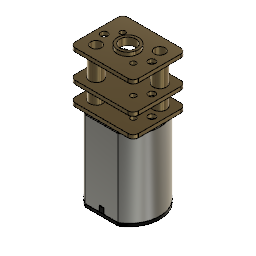
Semana4_Desafio2 v1 (Autodesk Fusion 360 design; units mm, degrees)
Autodesk Fusion 360 part; units mm, degrees
sketch "Sketch1" plane through (0, 0, 0) normal (0, 0, 1) x (1, 0, 0)
  line L0 (5, -5) -> (-5, -5)
  line L1 (-6, -4) -> (-6, 4)
  line L2 (-5, 5) -> (5, 5)
  line L3 (6, 4) -> (6, -4)
  line L4 (6, -5) -> (-6, 5) construction
  line L5 (-6, -5) -> (6, 5) construction
  circle A0 centre (0, 0) radius 2
  circle A1 centre (0, 0) radius 1.5
  circle A2 centre (-4.5, 0) radius 0.65
  circle A3 centre (4.5, 0) radius 0.65
  line L6 (-1.118, 1) -> (1.118, 1)
  arc A4 (-5, 5) -> (-6, 4) centre (-5, 4) ccw
  arc A5 (6, 4) -> (5, 5) centre (5, 4) ccw
  arc A6 (5, -5) -> (6, -4) centre (5, -4) ccw
  arc A7 (-6, -4) -> (-5, -5) centre (-5, -4) ccw
  point P0 (0, -1.5)
  dimension "d1" = 12
  dimension "d2" = 10
  dimension "d3" = 4
  dimension "d4" = 3
  dimension "d6" = 2.5
  dimension "d7" = 1.3
  dimension "d8" = 1.3
  dimension "d9" = 4.5
  dimension "d10" = 4.5
  dimension "d11" = 1
  dimension "d12" = 1
  dimension "d13" = 1
  dimension "d14" = 1
  constraint horizontal L0
  constraint perpendicular L0 L1
  constraint parallel L0 L2
  constraint parallel L1 L3
  constraint coincident L4 A0.centre
  constraint coincident L5 A0.centre
  constraint coincident A0.centre A1.centre
  constraint coincident A1 P0
  constraint coincident A1 L6.start
  constraint coincident A1 L6.end
  constraint horizontal L6
  constraint coincident L4.end L1
  constraint coincident L4.end L2
  constraint tangent L1 A4
  constraint tangent L2 A4
  constraint coincident L5.end L2
  constraint coincident L5.end L3
  constraint tangent L2 A5
  constraint tangent L3 A5
  constraint coincident L4.start L0
  constraint coincident L4.start L3
  constraint tangent L0 A6
  constraint tangent L3 A6
  constraint coincident L5.start L1
  constraint coincident L5.start L0
  constraint tangent L1 A7
  constraint tangent L0 A7
  measures "d1" distance of L4.end L5.end
  measures "d2" distance of L5.start L4.end
  measures "d3" diameter of A0
  measures "d4" diameter of A1
  measures "d6" distance of P0 L6
  measures "d7" diameter of A2
  measures "d8" diameter of A3
  measures "d9" distance of A0.centre A2.centre
  measures "d10" distance of A0.centre A3.centre
  measures "d11" radius of A4
  measures "d12" radius of A5
  measures "d13" radius of A6
  measures "d14" radius of A7
extrude "Extrude1" add sketch "Sketch1" along normal blind 0.7 contours L0 L1 L2 L3 A4 A5 A6 A7 makes body 1
extrude "Extrude2" add sketch "Sketch1" along normal blind 1.4 contours A0 bodies 1
ref_plane "WorkPlane1" through (0, 0, -9) normal (0, 0, 1) x (1, 0, 0)
sketch "Sketch2" plane through (0, 0, -9) normal (0, 0, 1) x (1, 0, 0)
  line L0 (-3.1, 5) -> (3.1, 5)
  line L1 (3.1, -5) -> (-3.1, -5)
  line L2 (-6, 5) -> (6, -5) construction
  line L3 (6, 5) -> (-6, -5) construction
  line L4 (0, -5) -> (3.1, -5) construction
  line L5 (0, -5) -> (-3.1, -5) construction
  line L6 (3.1, 5) -> (-3.1, 5) construction
  arc A0 (-3.1, 5) -> (-3.1, -5) centre (-0.2397, 0) ccw
  arc A1 (-3.1, 5) -> (-3.1, -5) centre (-0.2397, 0) ccw
  arc A2 (-2.9641, 4.5) -> (-2.9641, -4.5) centre (-0.2397, 0) ccw
  arc A3 (3.1, -5) -> (3.1, 5) centre (0.2397, 0) ccw
  arc A4 (2.9641, -4.5) -> (2.9641, 4.5) centre (0.2397, 0) ccw
  line L7 (-2.9641, 4.5) -> (2.9641, 4.5)
  line L8 (-2.9641, -4.5) -> (2.9641, -4.5)
  line L9 (5, -5) -> (-5, -5)
  dimension "d20" = 3.1
  dimension "d21" = 3.1
  dimension "d22" = 6.2
  dimension "d24" = 10.521
  dimension "d27" = 0.5
  dimension "d28" = 0.5
  constraint horizontal L0
  constraint parallel L0 L1
  constraint coincident L2 origin
  constraint coincident L3 origin
  constraint parallel L1 L4
  constraint parallel L1 L5
  constraint coincident L1 L4.start
  constraint horizontal L8
  measures "d20" distance of L4.start L1.end
  measures "d21" distance of L4.start L1.start
  measures "d22" distance of L0.end L0.start
  measures "d24" diameter of A2
  measures "d27" distance of L1 L8
  measures "d28" distance of L6 L7
extrude "Extrude3" add sketch "Sketch2" against normal blind 14.8 separate body makes body 2
sketch "Sketch3" plane through (0, 0, -9) normal (0, 0, 1) x (-1, 0, 0)
  arc A0 (2.9641, -4.5) -> (2.9641, 4.5) centre (0.2397, 0) ccw
  line L0 (2.9641, -4.5) -> (-2.9641, -4.5)
  arc A1 (-2.9641, 4.5) -> (-2.9641, -4.5) centre (-0.2397, 0) ccw
  line L1 (-2.9641, 4.5) -> (2.9641, 4.5)
  arc A2 (3.1, -5) -> (3.1, 5) centre (0.2397, 0) ccw
  line L2 (3.1, 5) -> (-3.1, 5)
  arc A3 (-3.1, 5) -> (-3.1, -5) centre (-0.2397, 0) ccw
  line L3 (-3.1, -5) -> (3.1, -5)
  arc A4 (-2.9641, 4.5) -> (-2.9641, -4.5) centre (-0.2397, 0) ccw
  arc A5 (2.9641, -4.5) -> (2.9641, 4.5) centre (0.2397, 0) ccw
  line L4 (2.9641, 4.5) -> (-2.9641, 4.5)
  line L5 (2.9641, -4.5) -> (-2.9641, -4.5)
  line L6 (5, 5) -> (-5, 5)
  line L7 (-6, 4) -> (-6, -4)
  line L8 (-5, -5) -> (5, -5)
  line L9 (6, -4) -> (6, 4)
  arc A6 (6, 4) -> (5, 5) centre (5, 4) ccw
  arc A7 (5, -5) -> (6, -4) centre (5, -4) ccw
  arc A8 (-5, 5) -> (-6, 4) centre (-5, 4) ccw
  arc A9 (-6, -4) -> (-5, -5) centre (-5, -4) ccw
  point P0 (6, 5)
  point P1 (-6, -5)
  dimension "d31" = 1
  dimension "d32" = 1
  dimension "d33" = 1
  dimension "d34" = 1
  constraint concentric A0 A5
  constraint concentric A1 A4
  constraint coincident A0.end L1.end
  constraint coincident A1.start L1.start
  constraint coincident A0.start L0.start
  constraint coincident L0.end A1.end
  constraint horizontal L6
  constraint vertical L7
  constraint horizontal L8
  constraint vertical L9
  constraint tangent L9 A6
  constraint tangent L6 A6
  constraint tangent L9 A7
  constraint tangent L8 A7
  constraint tangent L6 A8
  constraint tangent L7 A8
  constraint tangent L7 A9
  constraint tangent L8 A9
  measures "d31" radius of A6
  measures "d32" radius of A7
  measures "d33" radius of A8
  measures "d34" radius of A9
ref_plane "WorkPlane2" through (0, 0, -5.3) normal (0, 0, 1) x (1, 0, 0)
sketch "Sketch5" plane through (0, 0, -5.3) normal (0, 0, 1) x (1, 0, 0)
  line L0 (5, -5) -> (-5, -5)
  line L1 (-6, -4) -> (-6, 4)
  line L2 (-5, 5) -> (5, 5)
  line L3 (6, 4) -> (6, -4)
  line L4 (6, -5) -> (-6, 5) construction
  line L5 (-6, -5) -> (6, 5) construction
  arc A0 (-6, -4) -> (-5, -5) centre (-5, -4) ccw
  arc A1 (5, -5) -> (6, -4) centre (5, -4) ccw
  arc A2 (6, 4) -> (5, 5) centre (5, 4) ccw
  arc A3 (-5, 5) -> (-6, 4) centre (-5, 4) ccw
  dimension "d43" = 12
  dimension "d44" = 10
  dimension "d45" = 1
  dimension "d46" = 1
  dimension "d47" = 1
  dimension "d48" = 1
  constraint horizontal L0
  constraint perpendicular L0 L1
  constraint parallel L0 L2
  constraint parallel L1 L3
  constraint coincident L4 origin
  constraint coincident L5 origin
  constraint coincident L5.start L1
  constraint coincident L5.start L0
  constraint tangent L1 A0
  constraint tangent L0 A0
  constraint coincident L4.start L0
  constraint coincident L4.start L3
  constraint tangent L0 A1
  constraint tangent L3 A1
  constraint coincident L5.end L2
  constraint coincident L5.end L3
  constraint tangent L2 A2
  constraint tangent L3 A2
  constraint coincident L4.end L1
  constraint coincident L4.end L2
  constraint tangent L1 A3
  constraint tangent L2 A3
  measures "d43" distance of L4.end L5.end
  measures "d44" distance of L5.start L4.end
  measures "d45" radius of A0
  measures "d46" radius of A1
  measures "d47" radius of A2
  measures "d48" radius of A3
extrude "Extrude5" add sketch "Sketch5" along normal blind 0.7 separate body makes body 3
sketch "Sketch6" plane through (0, 0, 0.7) normal (0, 0, 1) x (-1, 0, 0)
  circle A0 centre (-4.5, 0) radius 0.65
  circle A1 centre (0, 0) radius 2
  circle A2 centre (4.5, 0) radius 0.65
  arc A3 (5, -5) -> (6, -4) centre (5, -4) ccw
  line L0 (6, -4) -> (6, 4)
  arc A4 (6, 4) -> (5, 5) centre (5, 4) ccw
  line L1 (5, 5) -> (-5, 5)
  arc A5 (-5, 5) -> (-6, 4) centre (-5, 4) ccw
  line L2 (-6, 4) -> (-6, -4)
  arc A6 (-6, -4) -> (-5, -5) centre (-5, -4) ccw
  line L3 (-5, -5) -> (5, -5)
  circle A7 centre (3.5, 2.5) radius 1.25
  circle A8 centre (-3.5, -2.5) radius 1.25
  line L4 (5, -5) -> (-5, -5)
  line L5 (-6, -4) -> (-6, 4)
  line L6 (-5, 5) -> (5, 5)
  line L7 (6, 4) -> (6, -4)
  circle A9 centre (-3, 2) radius 0.5
  circle A10 centre (3, -2) radius 0.5
  circle A11 centre (3.5, 2.5) radius 1
  circle A12 centre (-3.5, -2.5) radius 1
  dimension "d51" = 2.5
  dimension "d52" = 2.5
  dimension "d53" = 2.5
  dimension "d54" = 2.5
  dimension "d55" = 2.5
  dimension "d56" = 2.5
  dimension "d57" = 1
  dimension "d58" = 1
  dimension "d59" = 3
  dimension "d60" = 3
  dimension "d61" = 3
  dimension "d62" = 3
  dimension "d63" = 2
  dimension "d64" = 2
  constraint concentric A7 A11
  constraint concentric A8 A12
  measures "d51" diameter of A7
  measures "d52" diameter of A8
  measures "d53" distance of A8.centre L4
  measures "d54" distance of A8.centre L5
  measures "d55" distance of A7.centre L6
  measures "d56" distance of A7.centre L7
  measures "d57" diameter of A9
  measures "d58" diameter of A10
  measures "d59" distance of L4 A10.centre
  measures "d60" distance of L7 A10.centre
  measures "d61" distance of L6 A9.centre
  measures "d62" distance of L5 A9.centre
  measures "d63" diameter of A11
  measures "d64" diameter of A12
extrude "Extrude6" add sketch "Sketch6" against normal blind 9 contours A7 bodies 1 2 3
extrude "Extrude7" add sketch "Sketch6" against normal blind 9 contours A8 bodies 1 2
extrude "Extrude8" cut sketch "Sketch6" against normal blind 15 contours A9 | A10 | A11 | A12 bodies 1
fillet "Fillet1" radius 0.25 4 edges at (0, -5, -9) (6, 0, -9) (-6, 0, -9) (0, 5, -9) on bodies 2
extrude "Extrude9" add sketch "Sketch3" along normal blind 0.7 contours A0 L0 A1 L1 A4 A5 L4 L5 | A2 L2 A3 L3 L6 L8 | A2 L8 L9 A7 | A2 L6 L9 A6 | A3 L7 L8 A9 | A3 L6 L7 A8 bodies 1 2
sketch "Sketch7" plane through (0, 0, -23.8) normal (0, 0, -1) x (1, 0, 0)
  arc A0 (-2.9641, 4.5) -> (-2.9641, -4.5) centre (-0.2397, 0) ccw
  line L0 (-2.9641, 4.5) -> (2.9641, 4.5)
  arc A1 (2.9641, -4.5) -> (2.9641, 4.5) centre (0.2397, 0) ccw
  line L1 (2.9641, -4.5) -> (-2.9641, -4.5)
  arc A2 (-3.1, 5) -> (-3.1, -5) centre (-0.2397, 0) ccw
  line L2 (-3.1, -5) -> (3.1, -5)
  arc A3 (3.1, -5) -> (3.1, 5) centre (0.2397, 0) ccw
  line L3 (3.1, 5) -> (-3.1, 5)
  line L4 (0.4999, -5) -> (-0.4001, -5)
  line L5 (-0.4001, -4.5) -> (0.4999, -4.5)
  line L6 (0.4999, -5) -> (-0.4001, -5)
  line L7 (-0.4001, -4.5) -> (-0.4001, -5)
  line L8 (0.4999, -4.5) -> (0.4999, -5)
  line L9 (0.45, 4.5) -> (0.45, 5)
  line L10 (-0.45, 4.5) -> (0.45, 4.5)
  line L11 (-0.45, 5) -> (-0.45, 4.5)
  line L12 (-0.45, 5) -> (0.45, 5)
  line L13 (-0.4001, -4.5) -> (-2.9641, -4.5) construction
  line L14 (0.4999, -4.5) -> (2.9641, -4.5) construction
  line L15 (0.45, 4.5) -> (2.9641, 4.5) construction
  line L16 (-0.45, 4.5) -> (-2.9641, 4.5) construction
  line L17 (0, 0) -> (0.0499, -4.5) construction
  line L18 (0, 0) -> (0, 4.5) construction
  line L19 (0, 4.5) -> (-0.45, 4.5)
  dimension "d74" = 0.9
  dimension "d75" = 0.9
  constraint coincident L2 L4.start
  constraint coincident L2 L4.end
  constraint parallel L2 L4
  constraint coincident L1 L5.start
  constraint coincident L1 L5.end
  constraint parallel L1 L5
  constraint perpendicular L2 L7
  constraint perpendicular L2 L8
  constraint coincident L0 L9.start
  constraint coincident L3 L9.end
  constraint perpendicular L3 L9
  constraint coincident L0 L10.start
  constraint perpendicular L9 L10
  constraint coincident L3 L11.start
  constraint perpendicular L0 L11
  constraint coincident A0.end L1.end
  constraint coincident A1.start L1.start
  constraint coincident L0.end A1.end
  constraint coincident A0.start L0.start
  constraint coincident L17.start L18.start
  constraint midpoint L5 L17.end
  constraint midpoint L0 L18.end
  constraint midpoint L10 L18.end
  measures "d74" distance of L4.start L4.end
  measures "d75" distance of L9.end L11.start
extrude "Extrude10" cut sketch "Sketch7" against normal blind 1 contours L0 L3 L9 L10 L11 L12 L19 | L1 L2 L4 L5 L6 L7 L8 bodies 1
sketch "Sketch9" plane through (0, 0, -23.8) normal (0, 0, -1) x (1, 0, 0)
  line L0 (0.4999, -4.5) -> (0.4999, -5)
  line L1 (0.4999, -5) -> (3.1, -5)
  arc A0 (3.1, -5) -> (3.1, 5) centre (0.2397, 0) ccw
  line L2 (3.1, 5) -> (0.45, 5)
  line L3 (0.45, 5) -> (0.45, 4.5)
  line L4 (0.45, 4.5) -> (2.9641, 4.5)
  arc A1 (2.9641, -4.5) -> (2.9641, 4.5) centre (0.2397, 0) ccw
  line L5 (2.9641, -4.5) -> (0.4999, -4.5)
  arc A2 (3.1, -5) -> (3.1, 5) centre (0.2397, 0) ccw
  arc A3 (-3.1, 5) -> (-3.1, -5) centre (-0.2397, 0) ccw
  line L6 (3.1, 5) -> (-3.1, 5)
  line L7 (3.1, -5) -> (-3.1, -5)
  constraint coincident A0.end L2.start
  constraint coincident A3.start L6.end
  constraint coincident L1.end A0.start
  constraint coincident A3.end L7.end
extrude "Extrude11" add sketch "Sketch9" along normal blind 0.6 separate body makes body 4
sketch "Sketch12" plane through (0, 0, -24.4) normal (0, 0, -1) x (1, 0, 0)
  line L0 (3.1, 5) -> (-3.1, 5)
  arc A0 (-3.1, 5) -> (-3.1, -5) centre (-0.2397, 0) ccw
  line L1 (-3.1, -5) -> (3.1, -5)
  arc A1 (3.1, -5) -> (3.1, 5) centre (0.2397, 0) ccw
  line L2 (-0.4, 5) -> (0.4, 5)
  line L3 (0.4, 5) -> (0.4, 4.5)
  line L4 (0.4, 4.5) -> (-0.4, 4.5)
  line L5 (-0.4, 4.5) -> (-0.4, 5)
  line L6 (-0.4, -5) -> (0.4, -5)
  line L7 (0.4, -5) -> (0.4, -4.5)
  line L8 (0.4, -4.5) -> (-0.4, -4.5)
  line L9 (-0.4, -4.5) -> (-0.4, -5)
  line L10 (0, 0) -> (0, -4.5) construction
  line L11 (0, 0) -> (0, 4.5) construction
  dimension "d84" = 0.8
  dimension "d85" = 0.5
  dimension "d86" = 0.8
  dimension "d87" = 0.5
  constraint horizontal L2
  constraint vertical L3
  constraint horizontal L4
  constraint vertical L5
  constraint coincident L0 L2.start
  constraint horizontal L6
  constraint vertical L7
  constraint horizontal L8
  constraint vertical L9
  constraint collinear L1 L6
  constraint coincident L10.start L11.start
  constraint coincident L8 L10.end
  constraint perpendicular L8 L10
  constraint midpoint L8 L10.end
  constraint coincident L4 L11.end
  constraint perpendicular L4 L11
  constraint midpoint L4 L11.end
  measures "d84" distance of L2.start L2.end
  measures "d85" distance of L2.start L4.end
  measures "d86" distance of L6.start L6.end
  measures "d87" distance of L6.start L8.end
extrude "Extrude13" add sketch "Sketch12" against normal blind 1.7 contours L0 L2 L3 L4 L5 | L1 L6 L7 L8 L9 bodies 4
extrude "Extrude14" cut sketch "Sketch6" against normal blind 10 contours A0 | A2 bodies 1
extrude "Extrude15" cut sketch "Sketch6" against normal blind 10 contours A9 | A10 bodies 1
sketch "Sketch13" plane through (0, 0, -24.4) normal (0, 0, -1) x (1, 0, 0)
  line L0 (-3.1, -5) -> (3.1, -5)
  arc A0 (3.1, -5) -> (3.1, 5) centre (0.2397, 0) ccw
  line L1 (3.1, 5) -> (-3.1, 5)
  arc A1 (-3.1, 5) -> (-3.1, -5) centre (-0.2397, 0) ccw
  circle A2 centre (0, 0) radius 2.5
  circle A3 centre (0, 0) radius 0.5
  dimension "d96" = 5
  dimension "d97" = 1
  constraint coincident A2.centre A3.centre
  constraint concentric A2 A3
  measures "d96" diameter of A2
  measures "d97" diameter of A3
extrude "Extrude16" add sketch "Sketch13" along normal blind 0.8 separate body contours A2 makes body 5
ref_plane "WorkPlane3" through (0, -2.5, -24.8638) normal (0, -1, 0) x (1, 0, 0)
sketch "Sketch14" plane through (0, -2.5, -24.8638) normal (0, -1, 0) x (1, 0, 0)
  line L0 (-1, 0.4638) -> (1, 0.4638)
  line L1 (1, 0.4638) -> (1, -0.3365)
  line L2 (-1, 0.4638) -> (-1, -0.3362)
  circle A0 through (-2.5, 0.4638, -2.5) (1.25, 0.4638, -0.3349) (1.25, 0.4638, -4.6651) construction
  line L3 (0, 0.4638) -> (-1, 0.4638) construction
  line L4 (-1, 0.4638) -> (-1, -1.3362) construction
  line L5 (-1, -1.3362) -> (1, -1.3362) construction
  arc A1 (-1, -0.3362) -> (1, -0.3359) centre (0, -0.3362) ccw
  circle A2 centre (0, -0.3362) radius 0.5
  dimension "d101" = 2
  dimension "d102" = 1.8
  dimension "d103" = 1
  constraint perpendicular L0 L2
  constraint parallel L0 L3
  constraint collinear L0 L3
  constraint perpendicular L0 L4
  constraint perpendicular L4 L5
  constraint tangent L5 A1
  constraint tangent L4 A1
  constraint coincident A1 L1.end
  constraint coincident L1 A1.end
  constraint concentric A1 A2
  measures "d101" diameter of A1
  measures "d102" distance of L0.start L4.end
  measures "d103" diameter of A2
extrude "Extrude17" add sketch "Sketch14" along normal blind 0.25 bodies 4 5
ref_plane "WorkPlane4" through (0, 2.5, -24.6922) normal (0, 1, 0) x (-1, 0, 0)
sketch "Sketch15" plane through (0, 2.5, -24.6922) normal (0, 1, 0) x (1, 0, 0)
  circle A0 centre (0, 0.5) radius 0.5
  circle A1 through (-2.5, -0.2922, -2.5) (1.25, -0.2922, -0.3349) (1.25, -0.2922, -4.6651) construction
  line L0 (0, -0.2922) -> (-1.2, -0.2922) construction
  line L1 (-1, -0.2922) -> (-1, 0.5)
  line L2 (1, 0.5) -> (1, -0.3)
  line L3 (1, -0.3) -> (-1, -0.2922)
  arc A2 (1, 0.5) -> (-1, 0.5) centre (0, 0.5) ccw
  arc A3 (-0.6103, -0.2922) -> (-0.6083, -0.2937) centre (0, 0.5) ccw
  line L4 (0.6, 1.5) -> (-0.9, 1.5) construction
  dimension "d107" = 2
  dimension "d108" = 1
  constraint concentric A0 A2
  constraint horizontal L0
  constraint coincident L0 L1.start
  constraint vertical L1
  constraint vertical L2
  constraint tangent L2 A2
  constraint tangent L1 A2
  constraint coincident L3 A3.end
  constraint coincident L0 A3.start
  constraint concentric A2 A3
  constraint horizontal L4
  constraint tangent A2 L4
  measures "d107" diameter of A2
  measures "d108" diameter of A0
extrude "Extrude18" add sketch "Sketch15" along normal blind 0.25 contours L1 L3 A3 | L3 A2 A3 | L2 L3 A3 bodies 4
